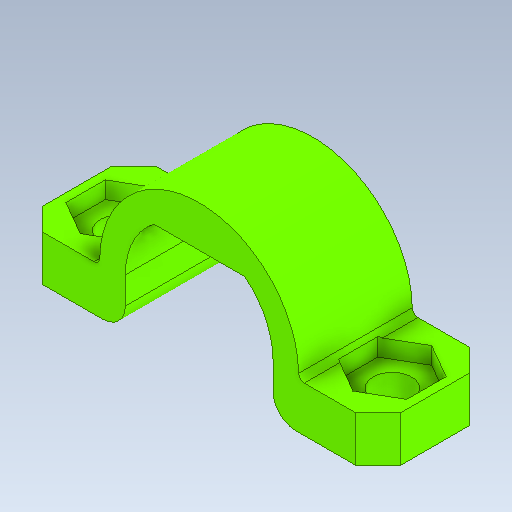
# Autodesk Inventor part: motor-clamp
Saved by Autodesk Inventor 2020 (Build 240168000, 168)
## iProperties
Created: 2020-11-03
Part Number: motor-clamp
Material: Generic
Document SubType Name: Modeling
Designer: alnwlsn
Density: 1 g/cm^3
Appearance: Default
Author: alnwlsn
Autodesk Inventor part; units mm, degrees
ref_plane "YZ Plane" through (0, 0, 0) normal (1, 0, 0) x (0, 1, 0)
ref_plane "XZ Plane" through (0, 0, 0) normal (0, 1, 0) x (-1, 0, 0)
ref_plane "XY Plane" through (0, 0, 0) normal (0, 0, 1) x (1, 0, 0)
sketch "Sketch1" plane through (0, 0, 0) normal (0, 0, 1) x (1, 0, 0)
  line L0 (0, 0) -> (7.25, 0)
  line L1 (0, 0) -> (0, 4)
  line L2 (0, 4) -> (6.5, 4)
  line L3 (9.25, 2) -> (9.25, 4.3765)
  arc A0 (11.75, 9.5) -> (9.25, 4.3765) centre (15.75, 4.3765) ccw
  arc A1 (7.25, 0) -> (9.25, 2) centre (7.25, 2) ccw
  line L4 (3.4828, -0.5) -> (32.44, -0.5) construction
  arc A2 (6.5, 4) -> (7, 4.4933) centre (6.5, 4.5) ccw
  line L5 (11.75, 9.5) -> (15.75, 9.5)
  line L6 (15.75, 9.5) -> (15.75, 6.4102) construction
  line L7 (15.75, 9.5) -> (19.75, 9.5)
  arc A3 (22.25, 4.3765) -> (19.75, 9.5) centre (15.75, 4.3765) ccw
  line L8 (22.25, 4.3765) -> (22.25, 2)
  arc A4 (22.25, 2) -> (24.25, 0) centre (24.25, 2) ccw
  line L9 (24.25, 0) -> (31.5, 0)
  line L10 (31.5, 0) -> (31.5, 4)
  line L11 (31.5, 4) -> (25, 4)
  arc A5 (24.5, 4.4933) -> (25, 4) centre (25, 4.5) ccw
  arc A6 (24.5, 4.4933) -> (7, 4.4933) centre (15.75, 4.3765) ccw
  line L12 (3.25, 4) -> (3.25, 2) construction
  line L13 (28.25, 4) -> (28.25, 2.1903) construction
  point P0 (6.9889, 4)
  dimension "d0" = 4
  dimension "d4" = 2
  dimension "d6" = 6.5
  dimension "d7" = 0.5
  dimension "d9" = 0.5
  dimension "d10" = 4
  dimension "d11" = 6.5
  dimension "d12" = 6.5
  dimension "d13" = 10
  dimension "d14" = 25
  constraints: 28 end point, 14 point on circle, 9 tangent, 7 centre point, 7 vertical, 5 equal length, 5 horizontal, 3 equal radius, 2 midpoint, 2 perpendicular, 1 collinear, 1 concentric, 1 point on line
  measures "d0" distance between parallel lines of L0 L2
  measures "d4" radius of A1
  measures "d6" radius of A0
  measures "d7" distance between parallel lines of L4 L0
  measures "d9" radius of A2
  measures "d10" distance of L5.start L5.end
  measures "d11" distance from line of L5.end L3
  measures "d12" distance of L1.end L2.end
  measures "d13" distance between parallel lines of L4 L7
  measures "d14" distance between parallel lines of L13 L12
extrude "Extrusion1" add sketch "Sketch1" along normal blind 10
chamfer "Chamfer1" distance 2 angle 45 4 edges at (0, 2, 10) (0, 2, 0) (31.5, 2, 10) (31.5, 2, 0)
sketch "Sketch2" plane through (6.5, 4, 10) normal (0, 1, 0) x (1, 0, 0)
  line L0 (-6.5, 8) -> (-6.5, 2) projected
  line L1 (-6.5, 5) -> (25, 5) construction
  line L2 (25, 8) -> (25, 2) projected
  circle A0 centre (-2.75, 5) radius 3.75 construction
  circle A1 centre (21.25, 5) radius 3.75 construction
  circle A2 centre (-2.75, 5) radius 1.7
  circle A3 centre (21.25, 5) radius 1.7
  line L3 (-2.75, 8.4641) -> (0.25, 6.7321)
  line L4 (0.25, 6.7321) -> (0.25, 3.2679)
  line L5 (0.25, 3.2679) -> (-2.75, 1.5359)
  line L6 (-2.75, 1.5359) -> (-5.75, 3.2679)
  line L7 (-5.75, 3.2679) -> (-5.75, 6.7321)
  line L8 (-5.75, 6.7321) -> (-2.75, 8.4641)
  line L9 (21.25, 8.4641) -> (24.25, 6.7321)
  line L10 (24.25, 6.7321) -> (24.25, 3.2679)
  line L11 (24.25, 3.2679) -> (21.25, 1.5359)
  line L12 (21.25, 1.5359) -> (18.25, 3.2679)
  line L13 (18.25, 3.2679) -> (18.25, 6.7321)
  line L14 (18.25, 6.7321) -> (21.25, 8.4641)
  point P0 (-6.5, 10)
  dimension "d20" = 24
  dimension "d21" = 3.4
  dimension "d22" = 6
  constraints: 26 end point, 4 centre point, 4 coincident, 2 equal radius, 2 midpoint, 2 point on line, 2 tangent, 2 vertical, 1 equal length, 26 other
  measures "d20" distance of A1.centre A0.centre
  measures "d21" diameter of A3
  measures "d22" distance between parallel lines of L11 L14
extrude "Extrusion2" cut sketch "Sketch2" along normal blind 10 contours A2 | A3 | L3 L4 L5 L6 L7 L8 | L9 L10 L11 L12 L13 L14
extrude "Extrusion3" cut sketch "Sketch2" against normal through all contours A2 | A3
extrude "Extrusion4" cut sketch "Sketch2" against normal blind 1.5 contours A2 | A3 | L3 L4 L5 L6 L7 L8 | L9 L10 L11 L12 L13 L14
body "Solid1"
